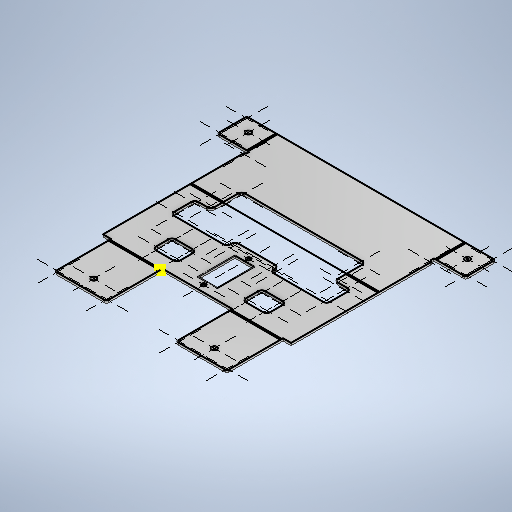
# Autodesk Inventor part: body_top_frame2_cam
Saved by Autodesk Inventor 2026.1 (Build 301233000, 233)
## iProperties
Created: 2026-02-06
Part Number: body_top_frame2_cam
Material: Aluminum 6061-AHC
Document SubType Name: Sheet Metal
Designer: chris
Density: 2.7 g/cm^3
Sheet Metal Rule: Default_mm
Appearance: Aluminum - Dark
Author: chris
Autodesk Inventor part; units mm, degrees
ref_plane "YZ Plane" through (0, 0, 0) normal (1, 0, 0) x (0, 1, 0)
ref_plane "XZ Plane" through (0, 0, 0) normal (0, 1, 0) x (-1, 0, 0)
ref_plane "XY Plane" through (0, 0, 0) normal (0, 0, 1) x (1, 0, 0)
sketch "Sketch1" plane through (0, 0, 0) normal (0, 1, 0) x (-1, 0, 0)
  line L0 (32, -0.4496) -> (0, -0.4496)
  line L1 (-80.1396, -91.6786) -> (-80.1396, -109.8686)
  line L2 (37, -56.2289) -> (-80, -56.2289)
  line L3 (-43.5, -0.4496) -> (-75, -0.4496)
  line L4 (37.1396, -109.8686) -> (37.1396, -91.6786)
  arc A0 (-60, -65.8686) -> (-58, -67.8686) centre (-58, -65.8686) ccw
  line L5 (15, -67.8686) -> (-58, -67.8686)
  arc A1 (15, -67.8686) -> (17, -65.8686) centre (15, -65.8686) ccw
  line L6 (17, -50.7793) -> (17, -65.8686)
  arc A2 (27, -35.7793) -> (25, -33.7793) centre (25, -35.7793) ccw
  line L7 (-6, -33.7793) -> (25, -33.7793)
  arc A3 (-6, -33.7793) -> (-8, -35.7793) centre (-6, -35.7793) ccw
  line L8 (-8, -36.7793) -> (-8, -35.7793)
  arc A4 (-10, -38.7793) -> (-8, -36.7793) centre (-10, -36.7793) ccw
  arc A5 (-35, -36.7793) -> (-33, -38.7793) centre (-33, -36.7793) ccw
  line L9 (-35, -35.7793) -> (-35, -36.7793)
  arc A6 (-35, -35.7793) -> (-37, -33.7793) centre (-37, -35.7793) ccw
  line L10 (-68, -33.7793) -> (-37, -33.7793)
  arc A7 (-68, -33.7793) -> (-70, -35.7793) centre (-68, -35.7793) ccw
  line L11 (-70, -46.7793) -> (-70, -35.7793)
  line L12 (-27.5, -31.2793) -> (-27.5, -8.2793)
  line L13 (-15.5, -31.2793) -> (-27.5, -31.2793)
  line L14 (-15.5, -8.2793) -> (-15.5, -31.2793)
  line L15 (-27.5, -8.2793) -> (-15.5, -8.2793)
  circle A8 centre (-21.5, -5.7793) radius 1.25
  circle A9 centre (-21.5, -33.7793) radius 1.25
  arc A10 (-1.04, -19.5193) -> (0.96, -21.5193) centre (0.96, -19.5193) ccw
  line L16 (11.96, -21.5193) -> (0.96, -21.5193)
  arc A11 (0.96, -9.5193) -> (-1.04, -11.5193) centre (0.96, -11.5193) ccw
  line L17 (-1.04, -19.5193) -> (-1.04, -11.5193)
  arc A12 (11.96, -21.5193) -> (13.96, -19.5193) centre (11.96, -19.5193) ccw
  line L18 (13.96, -11.5193) -> (13.96, -19.5193)
  arc A13 (13.96, -11.5193) -> (11.96, -9.5193) centre (11.96, -11.5193) ccw
  line L19 (0.96, -9.5193) -> (11.96, -9.5193)
  arc A14 (-43.96, -21.5193) -> (-41.96, -19.5193) centre (-43.96, -19.5193) ccw
  line L20 (-41.96, -11.5193) -> (-41.96, -19.5193)
  arc A15 (-56.96, -19.5193) -> (-54.96, -21.5193) centre (-54.96, -19.5193) ccw
  line L21 (-43.96, -21.5193) -> (-54.96, -21.5193)
  arc A16 (-41.96, -11.5193) -> (-43.96, -9.5193) centre (-43.96, -11.5193) ccw
  line L22 (-54.96, -9.5193) -> (-43.96, -9.5193)
  arc A17 (-54.96, -9.5193) -> (-56.96, -11.5193) centre (-54.96, -11.5193) ccw
  line L23 (-56.96, -19.5193) -> (-56.96, -11.5193)
  arc A18 (25, -48.7793) -> (27, -46.7793) centre (25, -46.7793) ccw
  line L24 (27, -35.7793) -> (27, -46.7793)
  arc A19 (19, -48.7793) -> (17, -50.7793) centre (19, -50.7793) ccw
  arc A20 (-60, -50.7793) -> (-62, -48.7793) centre (-62, -50.7793) ccw
  line L25 (-60, -65.8686) -> (-60, -50.7793)
  arc A21 (-70, -46.7793) -> (-68, -48.7793) centre (-68, -46.7793) ccw
  line L26 (-62, -48.7793) -> (-68, -48.7793)
  line L27 (25, -48.7793) -> (19, -48.7793)
  line L28 (-33, -38.7793) -> (-10, -38.7793)
  circle A22 centre (-59, 25.095) radius 1.55
  circle A23 centre (16, 25.095) radius 1.55
  circle A24 centre (-89.6843, -101.7736) radius 1.55
  circle A25 centre (46.6843, -101.7736) radius 1.55
  arc A26 (-80, -88.6786) -> (-79, -89.6786) centre (-79, -88.6786) ccw
  arc A27 (36, -89.6786) -> (37, -88.6786) centre (36, -88.6786) ccw
  line L29 (35.94, -89.6786) -> (36, -89.6786)
  arc A28 (55.7793, -92.6786) -> (54.7793, -91.6786) centre (54.7793, -92.6786) ccw
  arc A29 (54.7793, -109.8686) -> (55.7793, -108.8686) centre (54.7793, -108.8686) ccw
  line L30 (54.7793, -109.8686) -> (-97.7793, -109.8686)
  arc A30 (-98.7793, -108.8686) -> (-97.7793, -109.8686) centre (-97.7793, -108.8686) ccw
  arc A31 (-97.7793, -91.6786) -> (-98.7793, -92.6786) centre (-97.7793, -92.6786) ccw
  line L31 (-97.7793, -91.6786) -> (-78.94, -91.6786)
  arc A32 (1, 33.19) -> (0, 32.19) centre (1, 32.19) ccw
  arc A33 (32, 32.19) -> (31, 33.19) centre (31, 32.19) ccw
  arc A34 (-74, 33.19) -> (-75, 32.19) centre (-74, 32.19) ccw
  arc A35 (-43.5, 32.19) -> (-44.5, 33.19) centre (-44.5, 32.19) ccw
  line L32 (-43.5, 32.19) -> (-43.5, -1.6493)
  line L33 (-74, 33.19) -> (-44.5, 33.19)
  line L34 (-75, -1.6493) -> (-75, 32.19)
  line L35 (-75, -1.6493) -> (-80, -1.6493)
  line L36 (-80, -88.6786) -> (-80, -1.6493)
  line L37 (1, 33.19) -> (31, 33.19)
  line L38 (32, 32.19) -> (32, -1.6493)
  line L39 (37, -1.6493) -> (32, -1.6493)
  line L40 (0, -1.6493) -> (0, 32.19)
  line L41 (0, -1.6493) -> (-43.5, -1.6493)
  line L42 (37, -1.6493) -> (37, -88.6786)
  line L43 (-98.7793, -108.8686) -> (-98.7793, -92.6786)
  line L44 (55.7793, -92.6786) -> (55.7793, -108.8686)
  line L45 (35.94, -91.6786) -> (54.7793, -91.6786)
  line L46 (35.94, -91.6786) -> (35.94, -89.6786)
  line L47 (-79, -89.6786) -> (-78.94, -89.6786)
  line L48 (-78.94, -89.6786) -> (-78.94, -91.6786)
  line L49 (-80.5893, -109.8686) -> (-80.5893, -91.6786)
  line L50 (37.5893, -91.6786) -> (37.5893, -109.8686)
  line L51 (-79.69, -91.6786) -> (-79.69, -109.8686)
  line L52 (36.69, -109.8686) -> (36.69, -91.6786)
  line L53 (-75, 0) -> (-43.5, 0)
  line L54 (37, -56.6786) -> (17, -56.6786)
  line L55 (-60, -56.6786) -> (-80, -56.6786)
  line L56 (-43.5, -0.8993) -> (-75, -0.8993)
  line L57 (17, -55.7793) -> (37, -55.7793)
  line L58 (-80, -55.7793) -> (-60, -55.7793)
  line L59 (32, -0.8993) -> (0, -0.8993)
  line L60 (0, 0) -> (32, 0)
  point P0 (0, 0)
  constraints: 122 end point, 70 tangent, 60 point on circle, 36 centre point, 34 point on line, 33 horizontal, 32 equal radius, 28 perpendicular, 28 vertical, 26 parallel, 1 collinear, 181 other
extrude "Plate1" add sketch "Sketch1" against normal blind 1.5 contours L38 L59 L40 L0 | L0 L40 L60 L38 | L60 L40 A32 L37 A33 L38 | L38 L39 L42 L57 L6 A19 L27 A18 L24 A2 L7 A3 L8 A4 L28 A5 L9 A6 L10 A7 L11 A21 L26 A20 L25 L58 L36 L35 L34 L56 L32 L41 L40 L59 | L42 L2 L6 L57 | L56 L34 L3 L32 | L42 L54 L6 L2 | L3 L34 L53 L32 | L42 A27 L29 L46 L45 L52 L30 L51 L31 L48 L47 A26 L36 L55 L25 A0 L5 A1 L6 L54 | L53 L34 A34 L33 A35 L32 | L25 L55 L36 L2 | L2 L36 L58 L25 | L45 L4 L30 L52 | L45 L50 L30 L4 | L45 A28 L44 A29 L30 L50 | L30 L1 L31 L51 | L30 L49 L31 L1 | L30 A30 L43 A31 L31 L49
equation "\"d0\" = Thickness"
equation "\"BendReliefWidth\" = Thickness"
equation "\"BendReliefDepth\" = 0.5 * Thickness"
equation "\"CornerReliefSize\" = 4 * Thickness"
equation "\"MinimumRemnant\" = 2 * Thickness"
equation "\"TransitionRadius\" = BendRadius"
equation "\"JacobiRadiusSize\" = BendRadius"
equation "\"GapSize\" = Thickness"
equation "\"Thickness\" = 1.5"
equation "\"BendRadius\" = 0.31"
body "Solid1"
